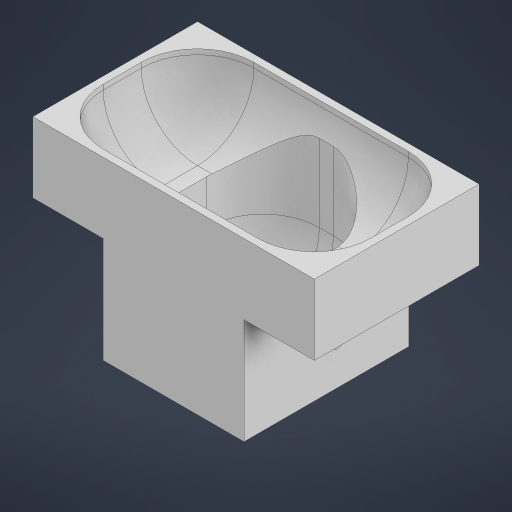
# Autodesk Inventor part: Part1
Saved by Autodesk Inventor 2023 (Build 270158000, 158)
## iProperties
Created: 2022-05-18
Part Number: Part1
Material: Generic
Document SubType Name: Modeling
Designer: jayso
Density: 1 g/cm^3
Appearance: Default
Author: jayso
Autodesk Inventor part; units mm, degrees
ref_plane "YZ Plane" through (0, 0, 0) normal (1, 0, 0) x (0, 1, 0)
ref_plane "XZ Plane" through (0, 0, 0) normal (0, 1, 0) x (-1, 0, 0)
ref_plane "XY Plane" through (0, 0, 0) normal (0, 0, 1) x (1, 0, 0)
sketch "Sketch1" plane through (0, 0, 0) normal (0, 1, 0) x (-1, 0, 0)
  point P0 (0, 0)
sketch "Sketch2" plane through (0, 0, 0) normal (0, 1, 0) x (-1, 0, 0)
  line L0 (50, -58.5) -> (-50, -58.5)
  line L1 (-50, -58.5) -> (-50, 58.5)
  line L2 (-50, 58.5) -> (50, 58.5)
  line L3 (50, 58.5) -> (50, -58.5)
  point P0 (0, 0)
  dimension "d0" = 100
  dimension "d1" = 117
  dimension "d2" = 50
  dimension "d3" = 58.5
  constraints: 8 end point, 2 parallel, 1 horizontal, 1 perpendicular
  measures "d0" distance of L0.start L0.end
  measures "d1" distance of L0.end L1.end
  measures "d2" distance from line of point (0, 0) L1
  measures "d3" distance from line of point (0, 0) L0
extrude "Extrusion1" add sketch "Sketch2" along normal blind 125
sketch "Sketch3" plane through (0, 125, 0) normal (0, 1, 0) x (1, 0, 0)
  line L0 (-45, 50) -> (45, 50)
  line L1 (45, 50) -> (45, -50)
  line L2 (45, -50) -> (-45, -50)
  line L3 (-45, -50) -> (-45, 50)
  line L4 (50, 58.5) -> (-50, 58.5) projected
  line L5 (-50, 58.5) -> (-50, -58.5) projected
  point P0 (0, 0)
  dimension "d6" = 90
  dimension "d7" = 100
  dimension "d8" = 8.5
  dimension "d9" = 5
  constraints: 8 end point, 2 parallel, 1 horizontal, 1 perpendicular
  measures "d6" distance of L0.end L0.start
  measures "d7" distance of L0.end L1.end
  measures "d8" distance between parallel lines of L4 L0
  measures "d9" distance between parallel lines of L5 L3
sketch "Sketch4" plane through (0, 0, 0) normal (0, -1, 0) x (1, 0, 0)
  line L0 (-45, 50) -> (45, 50)
  line L1 (45, 50) -> (45, -50)
  line L2 (45, -50) -> (-45, -50)
  line L3 (-45, -50) -> (-45, 50)
  line L4 (-50, 58.5) -> (50, 58.5) projected
  line L5 (-50, -58.5) -> (-50, 58.5) projected
  point P0 (0, 0)
  dimension "d10" = 90
  dimension "d11" = 100
  dimension "d12" = 8.5
  dimension "d13" = 5
  constraints: 8 end point, 2 parallel, 1 horizontal, 1 perpendicular
  measures "d10" distance of L0.start L0.end
  measures "d11" distance of L0.end L1.end
  measures "d12" distance between parallel lines of L4 L0
  measures "d13" distance between parallel lines of L5 L3
extrude "Extrusion2" add sketch "Sketch4" along normal blind 5
extrude "Extrusion3" cut sketch "Sketch3" against normal blind 115
sketch "Sketch6" plane through (-50, 0, -58.5) normal (-1, 0, 0) x (0, 0, 1)
  point P0 (58.5, 0)
sketch "Sketch7" plane through (-50, 0, -58.5) normal (-1, 0, 0) x (0, 0, 1)
  line L0 (0, 0) -> (0, 125) projected
  line L1 (117, 0) -> (117, 125) projected
  line L2 (0, 75) -> (117, 75)
  line L3 (117, 75) -> (117, 125)
  line L4 (117, 125) -> (0, 125)
  line L5 (0, 125) -> (0, 75)
  line L6 (0, 0) -> (117, 0) projected
  point P0 (58.5, 0)
  dimension "d23" = 75
  constraints: 8 end point, 2 parallel, 1 horizontal, 1 perpendicular, 1 point on line
  measures "d23" distance between parallel lines of L6 L2
extrude "Extrusion5" add sketch "Sketch7" along normal blind 50 contours L0 L4 L1 L2
sketch "Sketch8" plane through (50, 0, 58.5) normal (1, 0, 0) x (0, 0, -1)
  line L0 (0, 0) -> (0, 125) projected
  line L1 (117, 0) -> (117, 125) projected
  line L2 (0, 75) -> (117, 75)
  line L3 (117, 75) -> (117, 125)
  line L4 (117, 125) -> (0, 125)
  line L5 (0, 125) -> (0, 75)
  line L6 (0, 0) -> (117, 0) projected
  point P0 (58.5, 0)
  dimension "d26" = 75
  constraints: 8 end point, 2 parallel, 1 horizontal, 1 perpendicular, 1 point on line
  measures "d26" distance between parallel lines of L6 L2
extrude "Extrusion6" add sketch "Sketch8" along normal blind 50 contours L0 L4 L1 L2
sketch "Sketch9" plane through (0, 125, 0) normal (0, 1, 0) x (1, 0, 0)
  line L0 (94.7714, -53.5) -> (-95, -53.5)
  line L1 (-95, -53.5) -> (-95, 53.5)
  line L2 (-95, 53.5) -> (94.7714, 53.5)
  line L3 (94.7714, 53.5) -> (94.7714, -53.5)
  line L4 (100, -58.5) -> (-100, -58.5) projected
  line L5 (-100, 58.5) -> (100, 58.5) projected
  line L6 (-100, -58.5) -> (-100, 58.5) projected
  point P0 (0, 0)
  dimension "d29" = 5
  dimension "d30" = 5
  dimension "d31" = 5
  constraints: 8 end point, 2 parallel, 1 horizontal, 1 perpendicular
  measures "d29" distance between parallel lines of L4 L0
  measures "d30" distance between parallel lines of L5 L2
  measures "d31" distance between parallel lines of L6 L1
extrude "Extrusion7" cut sketch "Sketch9" against normal blind 43.65
fillet "Face Fillet1" radius 40 1 edges at (94.7714, 81.35, 0)
fillet "Face Fillet2" radius 40 1 edges at (-95, 81.35, 0)
fillet "Face Fillet3" radius 40 1 edges at (-0.1143, 81.35, -53.5)
fillet "Face Fillet4" radius 40 1 edges at (-0.1143, 81.35, 53.5)
sketch "Sketch11" plane through (0, -5, 0) normal (0, -1, 0) x (1, 0, 0)
  circle A0 centre (0, 37) radius 12
  line L0 (45, -50) -> (-45, -50) projected
  line L1 (-45, -13.5) -> (-45, 13.5) projected
  line L2 (45, 13.5) -> (45, 50) projected
  line L3 (45, 50) -> (-45, 50) projected
  point P0 (0, 0)
  dimension "d40" = 24
  dimension "d64" = 45
  dimension "d65" = 13
  constraints: 1 centre point
  measures "d40" diameter of A0
  measures "d64" distance from line of L2 A0.centre
  measures "d65" distance from line of L3 A0.centre
extrude "Extrusion8" cut sketch "Sketch11" against normal blind 43.65
sketch "Sketch12" plane through (50, 0, 58.5) normal (1, 0, 0) x (0, 0, -1)
  circle A0 centre (58.5, 37.5) radius 4
  line L0 (117, 0) -> (117, 75) projected
  line L1 (0, 75) -> (117, 75) projected
  point P0 (58.5, 0)
  point P1 (58.5, 75)
  dimension "d48" = 8
  dimension "d49" = 58.5
  dimension "d50" = 37.5
  constraints: 1 centre point, 1 midpoint
  measures "d48" diameter of A0
  measures "d49" distance from line of L0 A0.centre
  measures "d50" distance of point (58.5, 75) A0.centre
extrude "Extrusion9" add sketch "Sketch12" along normal blind 4
sketch "Sketch13" plane through (-50, 0, -58.5) normal (-1, 0, 0) x (0, 0, 1)
  circle A0 centre (58.5, 37.5) radius 4
  line L0 (0, 0) -> (117, 0) projected
  line L1 (117, 0) -> (117, 75) projected
  point P0 (58.5, 0)
  dimension "d53" = 8
  dimension "d54" = 37.5
  dimension "d55" = 58.5
  constraints: 1 centre point
  measures "d53" diameter of A0
  measures "d54" distance from line of L0 A0.centre
  measures "d55" distance from line of L1 A0.centre
extrude "Extrusion10" add sketch "Sketch13" along normal blind 4
sketch "Sketch14" plane through (-54, 37.5, 0) normal (-1, 0, 0) x (0, 0, 1)
  circle A0 centre (0, 0) radius 5.5
  point P0 (0, -37.5)
  dimension "d58" = 11
  constraints: 1 centre point
  measures "d58" diameter of A0
extrude "Extrusion11" add sketch "Sketch14" along normal blind 4
sketch "Sketch15" plane through (54, 37.5, 0) normal (1, 0, 0) x (0, 0, -1)
  circle A0 centre (0, 0) radius 4 projected
  circle A1 centre (0, 0) radius 5.5
  point P0 (0, -37.5)
  dimension "d61" = 11
  constraints: 1 centre point, 1 coincident
  measures "d61" diameter of A1
extrude "Extrusion12" add sketch "Sketch15" along normal blind 4 contours A0 | A1
fillet "Face Fillet8" radius 40 1 edges at (0, 10, -50)
fillet "Face Fillet9" radius 40 1 edges at (-45, 10, 20)
fillet "Face Fillet10" radius 40 1 edges at (45, 10, 20)
body "Solid1"
